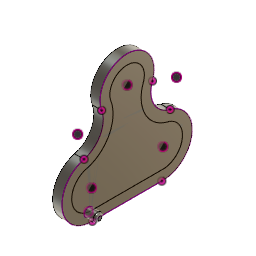
6.5 path pattern (Autodesk Fusion 360 design; units mm, degrees)
Autodesk Fusion 360 part; units mm, degrees
sketch "Sketch1" plane through (0, 0, 0) normal (1, 0, 0) x (0, 1, 0)
  line L0 (0, 0) -> (0, -99.0463) construction
  line L1 (-30.4057, -88.0396) -> (0, -88.0396)
  arc A0 (-37.6553, -37.4456) -> (-22.2115, -8.1006) centre (-43.2405, -15.7698) ccw
  arc A1 (-37.6553, -37.4456) -> (-30.4057, -88.0396) centre (-31.2401, -62.3428) ccw
  arc A2 (0, 23.6426) -> (-22.2115, -8.1006) centre (0, 0) ccw
  arc A3 (22.2115, -8.1006) -> (0, 23.6426) centre (0, 0) ccw
  line L2 (30.4057, -88.0396) -> (0, -88.0396)
  arc A4 (30.4057, -88.0396) -> (37.6553, -37.4456) centre (31.2401, -62.3428) ccw
  arc A5 (22.2115, -8.1006) -> (37.6553, -37.4456) centre (43.2405, -15.7698) ccw
  constraint coincident L0.start A2.centre
  constraint vertical L0
  constraint tangent A0 A2
  constraint tangent A0 A1
  constraint horizontal L1
  constraint coincident L0 L1.end
  constraint symmetric L0 L1.start L2.start
  constraint symmetric L0 A0.end A3.start
  constraint symmetric L0 A0.start A4.end
  constraint symmetric L0 A0 A5
  constraint symmetric L0 A1 A4
  constraint symmetric L0 A2 A3
  constraint symmetric L0 L1.end L2.end
  constraint symmetric L0 A2.start A3.end
extrude "Extrude1" add sketch "Sketch1" along normal blind 8.398
sketch "Sketch2" plane through (8.398, 0, 0) normal (1, 0, 0) x (0, 1, 0)
  circle A0 centre (-33.7553, -79.2573) radius 3.7955
extrude "Extrude2" add sketch "Sketch2" along normal blind 10
fillet "Fillet1" radius 2.082 1 edges at (18.398, -37.294, -80.6298)
sketch "Sketch3" plane through (8.398, 0, 0) normal (1, 0, 0) x (0, 1, 0)
  circle A0 centre (-33.7553, -79.2573) radius 3.7955
  arc A1 (22.2115, -8.1006) -> (-22.2115, -8.1006) centre (0, 0) ccw
  arc A2 (-37.6553, -37.4456) -> (-22.2115, -8.1006) centre (-43.2405, -15.7698) ccw
  arc A3 (-37.6553, -37.4456) -> (-30.4057, -88.0396) centre (-31.2401, -62.3428) ccw
  line L0 (-30.4057, -88.0396) -> (30.4057, -88.0396)
  arc A4 (30.4057, -88.0396) -> (37.6553, -37.4456) centre (31.2401, -62.3428) ccw
  arc A5 (22.2115, -8.1006) -> (37.6553, -37.4456) centre (43.2405, -15.7698) ccw
  arc A6 (14.1938, -5.1765) -> (-14.1938, -5.1765) centre (0, 0) ccw
  arc A7 (-35.5258, -45.7099) -> (-14.1938, -5.1765) centre (-43.2405, -15.7698) ccw
  arc A8 (-35.5258, -45.7099) -> (-30.5582, -79.5054) centre (-31.2401, -62.3428) ccw
  line L1 (-30.5582, -79.5054) -> (30.5582, -79.5054)
  arc A9 (30.5582, -79.5054) -> (35.5258, -45.7099) centre (31.2401, -62.3428) ccw
  arc A10 (14.1938, -5.1765) -> (35.5258, -45.7099) centre (43.2405, -15.7698) ccw
  dimension "d6" = 8.5343
